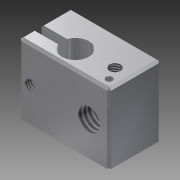
# Autodesk Inventor part: e3d_v6_heat_block
Saved by Autodesk Inventor 2013 (Build 170138000, 138)
## iProperties
Created: 2015-02-20
Part Number: e3d_v6_heat_block
Material: 一般
Document SubType Name: Modeling
Designer: Noa Izumi
Density: 1 g/cm^3
Author: Noa Izumi
Autodesk Inventor part; units mm, degrees
ref_plane "YZ Plane" through (0, 0, 0) normal (1, 0, 0) x (0, 1, 0)
ref_plane "XZ Plane" through (0, 0, 0) normal (0, 1, 0) x (-1, 0, 0)
ref_plane "XY Plane" through (0, 0, 0) normal (0, 0, 1) x (1, 0, 0)
sketch "草圖1" plane through (0, 0, 0) normal (0, 1, 0) x (-1, 0, 0)
  line L0 (0, 0) -> (20, 0)
  line L1 (20, 0) -> (20, 16)
  line L2 (20, 16) -> (0, 16)
  line L3 (0, 16) -> (0, 0)
  dimension "d0" = 20
  dimension "d1" = 16
  constraints: 8 end point, 2 parallel, 1 horizontal, 1 perpendicular
  measures "d0" distance of L0.start L0.end
  measures "d1" distance of L2.end L0.start
extrude "擠出1" add sketch "草圖1" along normal blind 11.5
sketch "草圖2" plane through (-20, 0, 16) normal (0, 0, 1) x (1, 0, 0)
  line L0 (0, 0) -> (20, 0) projected
  line L1 (20, 0) -> (20, 11.5) projected
  point P0 (16.5, 4.8)
  dimension "d4" = 3.5
  dimension "d5" = 4.8
  measures "d4" distance from line of L1 point (16.5, 4.8)
  measures "d5" distance from line of L0 point (16.5, 4.8)
hole "孔1" at (-3.5, 4.8, 16) direction (0, 0, -1) diameter 2.459 depth 3.5 tip angle 118 thread size "M3x0.5" class "6H" standard "ANSI Metric M Profile"
sketch "草圖3" plane through (-20, 0, 16) normal (0, 0, 1) x (1, 0, 0)
  line L0 (0, 0) -> (20, 0) projected
  line L1 (20, 0) -> (20, 11.5) projected
  point P0 (18, 2)
  dimension "d13" = 2
  dimension "d14" = 2
  measures "d13" distance from line of L1 point (18, 2)
  measures "d14" distance from line of L0 point (18, 2)
hole "孔2" at (-2, 2, 16) direction (0, 0, -1) diameter 1.5 depth 4.5 tip angle 118
chamfer "倒角1" distance 0.5 angle 45 12 edges at (-10, 0, 16) (0, 5.75, 16) (0, 0, 8) (-20, 0, 8) (-20, 5.75, 16) (0, 5.75, 0) (-10, 0, 0) (0, 11.5, 8) (-10, 11.5, 16) (-20, 11.5, 8) (-20, 5.75, 0) (-10, 11.5, 0)
sketch "草圖4" plane through (-19.5, 0.5, 16) normal (0, 0, 1) x (1, 0, 0)
  circle A0 centre (8, 3.5) radius 3
  line L0 (0, -0.5) -> (19, -0.5) projected
  line L1 (-0.5, 4.5) -> (8, 4.5)
  line L2 (8, 4.5) -> (8, 2.5)
  line L3 (8, 2.5) -> (-0.5, 2.5)
  line L4 (-0.5, 2.5) -> (-0.5, 4.5)
  point P0 (19.5, -0.5)
  dimension "d25" = 6
  dimension "d27" = 11.5
  dimension "d28" = 4
  dimension "d29" = 2
  dimension "d30" = 8.5
  constraints: 8 end point, 2 parallel, 1 centre point, 1 horizontal, 1 perpendicular
  measures "d25" diameter of A0
  measures "d27" horizontal distance of point (19.5, -0.5) A0.centre
  measures "d28" distance from line of L0 A0.centre
  measures "d29" distance of L3.end L1.start
  measures "d30" distance of L1.start L1.end
extrude "擠出2" cut sketch "草圖4" against normal through all
sketch "草圖5" plane through (0, 0, 0) normal (0, -1, 0) x (1, 0, 0)
  point P0 (0, 0)
  point P1 (-17.5, 8)
  dimension "d35" = 17.5
  measures "d35" horizontal distance of point (0, 0) point (-17.5, 8)
hole "孔3" at (-17.5, 0, 8) direction (0, 1, 0) diameter 2.459 end through all thread size "M3x0.5" class "6H" standard "ANSI Metric M Profile"
sketch "草圖6" plane through (0, 0, 0) normal (0, -1, 0) x (1, 0, 0)
  point P0 (0, 0)
  point P1 (-4.5, 8)
  dimension "d43" = 4.5
  measures "d43" horizontal distance of point (0, 0) point (-4.5, 8)
hole "孔4" at (-4.5, 0, 8) direction (0, 1, 0) diameter 4.917 end through all thread size "M6x1" class "6H" standard "ANSI Metric M Profile"
